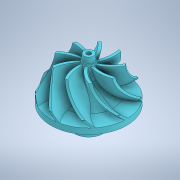
# Autodesk Inventor part: 40mm Impeller
Saved by Autodesk Inventor 2022 (Build 260153000, 153)
## iProperties
Created: 2023-01-14
Part Number: 40mm Impeller
Material: Generic
Document SubType Name: Modeling
Designer: ASUS
Density: 1 g/cm^3
Appearance: Cadet Blue
Author: ASUS
Autodesk Inventor part; units mm, degrees
ref_plane "YZ Plane" through (0, 0, 0) normal (1, 0, 0) x (0, 1, 0)
sketch "Sketch1" plane through (0, 0, 0) normal (1, 0, 0) x (0, 1, 0)
  line L0 (0, 0) -> (0, 20)
  line L1 (0, 0) -> (4.9015, 0)
  line L2 (0, 0) -> (20, 0)
  line L3 (20, 0) -> (20, 3)
  line L4 (0, 20) -> (3, 20)
  line L5 (3, 20) -> (6, 6)
  line L6 (6, 6) -> (20, 3)
  arc A0 (4.5, 13) -> (13, 4.5) centre (15.3182, 15.3182) ccw
  line L7 (0, 0) -> (22.4424, 0) construction
  dimension "d0" = 20
  dimension "d1" = 0
  dimension "d2" = 20
  dimension "d3" = 3
  dimension "d4" = 3
  dimension "d5" = 7
  dimension "d6" = 7
  dimension "d7" = 0
  constraints: 16 end point, 3 horizontal, 2 midpoint, 2 point on circle, 1 centre point, 1 equal length, 1 perpendicular, 1 tangent, 1 vertical
  measures "d0" distance of L0.start L0.end
  measures "d1" distance of L0.start L7.start
  measures "d2" distance of L0.start L2.end
  measures "d3" distance of L2.end L3.end
  measures "d4" distance of L0.end L4.end
  measures "d5" horizontal distance of L5.end A0.end
  measures "d6" vertical distance of L5.end A0.start
  measures "d7" distance from line of L7.start L0
revolve "Revolution1" add sketch "Sketch1" angle 360 about axis through (0, 0, 0) along (0, 1, 0)
ref_plane "Work Plane1" through (0, 19, 0) normal (0, 1, 0) x (1, 0, 0)
sketch "Sketch3" plane through (0, 19, 0) normal (0, 1, 0) x (1, 0, 0)
  line L0 (0, 0) -> (0, 27.3283) construction
  circle A0 centre (0, 0) radius 1.75 projected
  circle A1 centre (0, 0) radius 20 projected
  line L1 (0, 0) -> (-12.8558, 15.3209) construction
  arc A2 (0, 0) -> (-12.8558, 15.3209) centre (-15.5572, 0) ccw construction
  arc A3 (0.625, 0) -> (-12.3708, 15.7151) centre (-16.2766, -0.7459) ccw
  arc A4 (-0.625, 0) -> (-13.3282, 14.9117) centre (-17.4773, -1.4896) ccw
  arc A5 (-12.3708, 15.7151) -> (-13.3282, 14.9117) centre (0, 0) ccw
  line L2 (-0.625, 0) -> (0.625, 0)
  dimension "d14" = 40
  dimension "d15" = 0.625
  dimension "d16" = 0.625
  dimension "d17" = 16.918
  dimension "d18" = 16.918
  dimension "d19" = 0.625
  dimension "d20" = 0.625
  constraints: 12 point on circle, 6 end point, 4 centre point, 1 horizontal, 1 tangent, 1 vertical
  measures "d14" angle of L0 L1
  measures "d15" distance of L0.start L2.start
  measures "d16" distance of L0.start L2.end
  measures "d17" radius of A4
  measures "d18" radius of A3
  measures "d19" distance of L1.end A1.end
  measures "d20" distance of L1.end A4.end
ref_plane "Work Plane2" through (-12.8558, 19, -15.3209) normal (-0.6428, 0, -0.766) x (0, -1, 0)
sketch "Sketch4" plane through (-12.8558, 19, -15.3209) normal (-0.6428, 0, -0.766) x (0, -1, 0)
  line L0 (0, 0) -> (3.4115, 0.3507) construction
  line L1 (3.4115, 0.3507) -> (8.81, 3.2218) construction
  line L2 (8.81, 3.2218) -> (14.3158, 8.0668) construction
  line L3 (14.3158, 8.0668) -> (16.3894, 14.5626) construction
  line L4 (19, 20) -> (19, -20) projected
  line L5 (16.3894, 14.5626) -> (19, 15.3454) construction
  spline S0 degree 4 poles (0, 0) (3.4115, 0.3507) (8.81, 3.2218) (14.3158, 8.0668) (16.3894, 14.5626) (19, 15.3454) knots 1 1 1 1 1 2 3 3 3 3 3
  point P0 (19, 0)
  constraints: 1 point on line, 3 other
sweep "Sweep1" add profiles "Sketch3" path "Sketch4" picked at (-0.136, 1.2979) picked at (-2.7852, 7.6386) path curves S0 contours A3 L2 A4 A0 | A0 A4 A1 A3
pattern_circular "Circular Pattern1" count 9 over 360 about axis through (0, -10, 0) along (0, 1, 0) of "Sweep1"
sketch "Sketch5" plane through (0, 0, 0) normal (0, 0, 1) x (1, 0, 0)
  line L0 (20, 0) -> (17.6147, 0) projected
  line L1 (20, 0) -> (20, 6.5)
  line L2 (0, 20) -> (10, 20)
  line L3 (10, 20) -> (14, 20)
  line L4 (14, 20) -> (20, 20)
  line L5 (20, 20) -> (20, 6.5)
  line L6 (20, 20) -> (29.6294, 20)
  line L7 (29.6294, 20) -> (29.6294, -4.1299)
  line L8 (29.6294, -4.1299) -> (20, -4.1299)
  line L9 (20, -4.1299) -> (20, 20)
  line L10 (20, -4.1299) -> (0, -4.1299)
  line L11 (0, -4.1299) -> (0, 0)
  line L12 (0, 0) -> (20, 0)
  line L13 (20, 0) -> (20, -4.1299)
  line L14 (0, -8.9559) -> (0, 24.826) projected
  line L15 (3, 20) -> (-3, 20) projected
  line L16 (14, 20) -> (14, 12.4892) construction
  arc A0 (13.8, 20) -> (19.866, 6.3515) centre (32.1875, 20) ccw
  line L17 (19.866, 6.3515) -> (20, 6.2317)
  point P0 (19.8544, 0)
  dimension "d26" = 6.5
  dimension "d27" = 10
  dimension "d28" = 4
  dimension "d47" = 0
  dimension "d48" = 0
  constraints: 30 end point, 4 parallel, 3 horizontal, 3 perpendicular, 2 point on circle, 2 point on line, 2 vertical, 1 centre point
  measures "d26" distance of L0.start L1.end
  measures "d27" distance of L2.start L2.end
  measures "d28" distance of L2.end L3.end
  measures "d47" distance from line of L14 L2.start
  measures "d48" distance between parallel lines of L15 L2
revolve "Revolution2" cut sketch "Sketch5" angle 360 about axis through (0, -10, 0) along (0, 1, 0) contours L9 L10 L11 L12 L0 | L1 L5 L6 L7 L8 L9 | L17 A0 L3 L4 L5 L1
sketch "Sketch6" plane through (0, 0, 0) normal (0, -1, 0) x (1, 0, 0)
  circle A0 centre (0, 0) radius 7.5
  dimension "d34" = 15
  constraints: 1 centre point, 1 coincident
  measures "d34" diameter of A0
extrude "Extrusion2" add sketch "Sketch6" along normal blind 10
sketch "Sketch7" plane through (0, 20, 0) normal (0, 1, 0) x (1, 0, 0)
  circle A0 centre (0, 0) radius 2.5
  dimension "d37" = 5
  constraints: 1 centre point, 1 coincident
  measures "d37" diameter of A0
extrude "Extrusion3" add sketch "Sketch7" along normal blind 3
sketch "Sketch8" plane through (0, -10, 0) normal (0, -1, 0) x (1, 0, 0)
  circle A0 centre (0, 0) radius 1.2
  dimension "d40" = 2.4
  constraints: 1 centre point, 1 coincident
  measures "d40" diameter of A0
extrude "Extrusion4" cut sketch "Sketch8" against normal blind 35
sketch "Sketch9" plane through (0, 0, 0) normal (0, 0, 1) x (1, 0, 0)
  circle A0 centre (0, -7.5) radius 1.4
  line L0 (1.2, -10) -> (-1.2, -10) projected
  point P0 (0, 0)
  dimension "d43" = 2.8
  dimension "d44" = 2.5
  constraints: 1 centre point
  measures "d43" diameter of A0
  measures "d44" distance from line of L0 A0.centre
extrude "Extrusion5" cut sketch "Sketch9" along normal through all both and the other way through all
body "Solid1"
